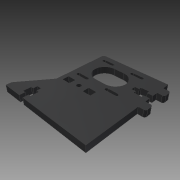
# Autodesk Inventor part: y_motor_mount
Saved by Autodesk Inventor 2014 (Build 180170000, 170)
## iProperties
Created: 2013-12-07
Part Number: y_motor_mount
Material: Plywood, Finish
Document SubType Name: Modeling
Designer: buben
Density: 0.552 g/cm^3
Appearance: Plywood - New
Author: buben
Subject: Laser Cutted
Autodesk Inventor part; units mm, degrees
ref_plane "YZ Plane" through (0, 0, 0) normal (1, 0, 0) x (0, 1, 0)
ref_plane "XZ Plane" through (0, 0, 0) normal (0, 1, 0) x (-1, 0, 0)
ref_plane "XY Plane" through (0, 0, 0) normal (0, 0, 1) x (1, 0, 0)
sketch "Sketch1" plane through (0, 0, 0) normal (0, 0, 1) x (1, 0, 0)
  line L0 (0, 0) -> (67.3, 0)
  line L1 (67.3, 0) -> (67.3, 55.5)
  line L2 (67.3, 55.5) -> (0, 55.5)
  line L3 (0, 55.5) -> (0, 0)
  line L4 (7, 48.5) -> (38, 48.5) construction
  line L5 (38, 48.5) -> (38, 17.5) construction
  line L6 (38, 17.5) -> (7, 17.5) construction
  line L7 (7, 17.5) -> (7, 48.5) construction
  line L8 (7, 48.5) -> (17, 48.5) construction
  line L9 (7, 50.1) -> (17, 50.1)
  line L10 (17, 46.9) -> (7, 46.9)
  arc A0 (7, 50.1) -> (7, 46.9) centre (7, 48.5) ccw
  arc A1 (17, 46.9) -> (17, 50.1) centre (17, 48.5) ccw
  line L11 (7, 17.5) -> (17, 17.5) construction
  line L12 (7, 19.1) -> (17, 19.1)
  line L13 (17, 15.9) -> (7, 15.9)
  arc A2 (7, 19.1) -> (7, 15.9) centre (7, 17.5) ccw
  arc A3 (17, 15.9) -> (17, 19.1) centre (17, 17.5) ccw
  line L14 (38, 48.5) -> (48, 48.5) construction
  line L15 (38, 46.9) -> (48, 46.9)
  line L16 (48, 50.1) -> (38, 50.1)
  arc A4 (38, 50.1) -> (38, 46.9) centre (38, 48.5) ccw
  arc A5 (48, 46.9) -> (48, 50.1) centre (48, 48.5) ccw
  line L17 (38, 17.5) -> (48, 17.5) construction
  line L18 (38, 19.1) -> (48, 19.1)
  line L19 (48, 15.9) -> (38, 15.9)
  arc A6 (38, 19.1) -> (38, 15.9) centre (38, 17.5) ccw
  arc A7 (48, 15.9) -> (48, 19.1) centre (48, 17.5) ccw
  line L20 (22.5, 33) -> (32.5, 33) construction
  line L21 (22.5, 44.5) -> (32.5, 44.5)
  line L22 (32.5, 21.5) -> (22.5, 21.5)
  arc A8 (22.5, 44.5) -> (22.5, 21.5) centre (22.5, 33) ccw
  arc A9 (32.5, 21.5) -> (32.5, 44.5) centre (32.5, 33) ccw
  point P0 (12, 48.5)
  point P1 (12, 17.5)
  point P2 (43, 48.5)
  point P3 (43, 17.5)
  point P4 (27.5, 33)
  point P5 (22.5, 48.5)
  point P6 (7, 33)
  dimension "d0" = 31
  dimension "d2" = 10
  dimension "d3" = 3.2
  dimension "d4" = 10
  dimension "d5" = 23
  dimension "d6" = 7
  dimension "d7" = 7
  dimension "d8" = 17.5
  dimension "d9" = 34.8
  constraints: 56 end point, 20 point on circle, 20 tangent, 14 parallel, 10 centre point, 7 midpoint, 6 coincident, 4 equal length, 3 equal radius, 3 horizontal alignment, 2 horizontal, 2 perpendicular, 1 vertical alignment
  measures "d0" distance of L5.end L6.end
  measures "d2" distance of L11.start L11.end
  measures "d3" distance between parallel lines of L13 L12
  measures "d4" distance of L20.start L20.end
  measures "d5" distance between parallel lines of L22 L21
  measures "d6" distance between parallel lines of L8 L2
  measures "d7" distance between parallel lines of L3 L7
  measures "d8" distance between parallel lines of L0 L6
  measures "d9" distance from line of L20.end L1
extrude "Extrusion1" add sketch "Sketch1" along normal blind 6.5
sketch "Sketch2" plane through (0, 0, 6.5) normal (0, 0, 1) x (1, 0, 0)
  line L0 (0, 0) -> (67.3, 0) projected
  line L1 (0, 55.5) -> (0, 0) projected
  line L2 (4, 9.5) -> (12, 9.5)
  line L3 (12, 9.5) -> (12, 3)
  line L4 (12, 3) -> (4, 3)
  line L5 (4, 3) -> (4, 9.5)
  line L6 (27, 9.5) -> (35, 9.5)
  line L7 (35, 9.5) -> (35, 3)
  line L8 (35, 3) -> (27, 3)
  line L9 (27, 3) -> (27, 9.5)
  line L10 (12, 3) -> (27, 9.5) construction
  line L11 (27, 3) -> (12, 9.5) construction
  circle A0 centre (19.5, 6.25) radius 2.25
  dimension "d12" = 8
  dimension "d13" = 6.5
  dimension "d14" = 15
  dimension "d15" = 4.5
  dimension "d16" = 3
  dimension "d17" = 4
  dimension "d18" = 8
  constraints: 20 end point, 4 parallel, 2 collinear, 2 horizontal, 2 perpendicular, 1 centre point, 1 midpoint
  measures "d12" distance of L2.start L2.end
  measures "d13" distance of L4.end L2.start
  measures "d14" distance between parallel lines of L9 L3
  measures "d15" diameter of A0
  measures "d16" distance between parallel lines of L0 L4
  measures "d17" distance between parallel lines of L1 L5
  measures "d18" distance of L6.start L6.end
extrude "Extrusion2" cut sketch "Sketch2" against normal through all
sketch "Sketch3" plane through (0, 0, 6.5) normal (0, 0, 1) x (1, 0, 0)
  arc A0 (32.5, 21.5) -> (32.5, 44.5) centre (32.5, 33) ccw projected
  line L0 (67.3, 0) -> (67.3, 55.5) projected
  line L1 (67.3, 35.25) -> (67.3, 30.75)
  line L2 (51, 30.75) -> (51, 35.25)
  line L3 (55, 37.75) -> (62.3, 37.75)
  line L4 (62.3, 28.25) -> (55, 28.25)
  line L5 (51, 35.25) -> (55, 35.25)
  line L6 (62.3, 35.25) -> (67.3, 35.25)
  line L7 (67.3, 30.75) -> (62.3, 30.75)
  line L8 (55, 30.75) -> (51, 30.75)
  line L9 (55, 28.25) -> (55, 30.75)
  line L10 (55, 35.25) -> (55, 37.75)
  line L11 (62.3, 37.75) -> (62.3, 35.25)
  line L12 (62.3, 30.75) -> (62.3, 28.25)
  point P0 (51, 33)
  dimension "d21" = 4.5
  dimension "d22" = 4
  dimension "d23" = 5
  dimension "d24" = 7.3
  dimension "d25" = 2.5
  dimension "d26" = 2.5
  constraints: 24 end point, 10 parallel, 5 collinear, 4 perpendicular, 3 horizontal, 1 horizontal alignment, 1 midpoint
  measures "d21" distance of L2.start L2.end
  measures "d22" distance of L2.end L5.end
  measures "d23" distance of L6.start L1.start
  measures "d24" distance of L3.start L3.end
  measures "d25" distance of L5.end L3.start
  measures "d26" distance of L4.end L8.start
extrude "Extrusion3" cut sketch "Sketch3" against normal through all
sketch "Sketch4" plane through (0, 0, 6.5) normal (0, 0, 1) x (1, 0, 0)
  line L0 (67.3, 35.25) -> (67.3, 55.5) projected
  line L1 (67.3, 0) -> (67.3, 30.75) projected
  line L2 (51, 30.75) -> (51, 35.25) projected
  line L3 (67.3, 40.5) -> (71.8, 40.5)
  line L4 (73.8, 42.5) -> (73.8, 46.5)
  line L5 (71.8, 48.5) -> (67.3, 48.5)
  line L6 (67.3, 48.5) -> (67.3, 40.5)
  line L7 (67.3, 25.5) -> (71.8, 25.5)
  line L8 (73.8, 23.5) -> (73.8, 19.5)
  line L9 (71.8, 17.5) -> (67.3, 17.5)
  line L10 (67.3, 17.5) -> (67.3, 25.5)
  arc A0 (73.8, 46.5) -> (71.8, 48.5) centre (71.8, 46.5) ccw
  arc A1 (71.8, 40.5) -> (73.8, 42.5) centre (71.8, 42.5) ccw
  arc A2 (73.8, 23.5) -> (71.8, 25.5) centre (71.8, 23.5) ccw
  arc A3 (71.8, 17.5) -> (73.8, 19.5) centre (71.8, 19.5) ccw
  point P0 (51, 33)
  dimension "d29" = 2
  dimension "d30" = 8
  dimension "d31" = 8
  dimension "d32" = 6.5
  dimension "d33" = 15
  dimension "d34" = 7.5
  constraints: 16 end point, 8 point on circle, 8 tangent, 4 centre point, 4 parallel, 3 equal radius, 2 horizontal, 2 perpendicular, 2 point on line, 1 collinear, 1 midpoint
  measures "d29" radius of A0
  measures "d30" distance between parallel lines of L5 L3
  measures "d31" distance between parallel lines of L9 L7
  measures "d32" distance between parallel lines of L0 L4
  measures "d33" distance between parallel lines of L7 L3
  measures "d34" distance from line of point (51, 33) L3
extrude "Extrusion4" add sketch "Sketch4" against normal blind 6.5
chamfer "Chamfer1" distance 2 angle 45 1 edges at (0, 55.5, 3.25)
sketch "Sketch5" plane through (0, 0, 6.5) normal (0, 0, 1) x (1, 0, 0)
  line L0 (7, 50.1) -> (17, 50.1) projected
  line L1 (-20.7, -32.99) -> (67.3, -32.99)
  line L2 (67.3, -32.99) -> (67.3, 0)
  line L3 (0, 0) -> (67.3, 0)
  line L4 (-20.7, -32.99) -> (-20.7, -27.99)
  line L5 (-20.7, -27.99) -> (0, 0)
  point P0 (67.3, 55.5)
  dimension "d40" = 88.49
  dimension "d41" = 88
  dimension "d42" = 5
  constraints: 10 end point, 3 perpendicular, 1 parallel
  measures "d40" distance of point (67.3, 55.5) L1.end
  measures "d41" distance of L1.start L1.end
  measures "d42" distance of L1.start L4.end
extrude "Extrusion5" add sketch "Sketch5" against normal blind 6.5
sketch "Sketch6" plane through (0, 0, 6.5) normal (0, 0, 1) x (1, 0, 0)
  line L0 (-20.7, -32.99) -> (67.3, -32.99) projected
  line L1 (-2.25, -16.69) -> (2.25, -16.69)
  line L2 (2.25, -32.99) -> (-2.25, -32.99)
  line L3 (4.75, -20.69) -> (4.75, -27.99)
  line L4 (-4.75, -27.99) -> (-4.75, -20.69)
  line L5 (-4.75, -20.69) -> (-2.25, -20.69)
  line L6 (2.25, -20.69) -> (4.75, -20.69)
  line L7 (4.75, -27.99) -> (2.25, -27.99)
  line L8 (-2.25, -27.99) -> (-4.75, -27.99)
  line L9 (-2.25, -32.99) -> (-2.25, -27.99)
  line L10 (-2.25, -20.69) -> (-2.25, -16.69)
  line L11 (2.25, -16.69) -> (2.25, -20.69)
  line L12 (2.25, -27.99) -> (2.25, -32.99)
  point P0 (0, 0)
  point P1 (0, -16.69)
  dimension "d45" = 4.5
  dimension "d46" = 2.5
  dimension "d47" = 2.5
  dimension "d48" = 5
  dimension "d49" = 4
  dimension "d50" = 7.3
  constraints: 24 end point, 10 parallel, 5 collinear, 4 perpendicular, 3 horizontal, 1 midpoint, 1 vertical alignment
  measures "d45" distance of L1.start L1.end
  measures "d46" distance of L4.end L5.end
  measures "d47" distance of L6.start L3.start
  measures "d48" distance of L2.end L8.start
  measures "d49" distance of L5.end L1.start
  measures "d50" distance of L4.start L4.end
extrude "Extrusion6" cut sketch "Sketch6" against normal through all
body "Solid1"
